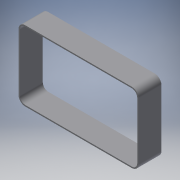
# Autodesk Inventor part: Hub Enclosure Back
Saved by Autodesk Inventor 2018 (Build 220112000, 112)
## iProperties
Created: 2018-03-25
Part Number: Hub Enclosure Back
Material: Generic
Document SubType Name: Modeling
Designer: brutu
Density: 1 g/cm^3
Appearance: Default
Author: brutu
Autodesk Inventor part; units mm, degrees
ref_plane "YZ Plane" through (0, 0, 0) normal (1, 0, 0) x (0, 1, 0)
ref_plane "XZ Plane" through (0, 0, 0) normal (0, 1, 0) x (-1, 0, 0)
ref_plane "XY Plane" through (0, 0, 0) normal (0, 0, 1) x (1, 0, 0)
sketch "Sketch1" plane through (0, 0, 0) normal (0, 0, 1) x (1, 0, 0)
  circle A0 centre (63.1, -31.85) radius 1.905 projected
  circle A1 centre (-63.1, -31.85) radius 1.905 projected
  arc A2 (-66.905, 25.805) -> (-54.205, 38.505) centre (-66.905, 38.505) ccw projected
  line L0 (-54.205, 38.505) -> (-54.205, 51.205) projected
  line L1 (-54.205, 51.205) -> (54.205, 51.205) projected
  line L2 (54.205, 51.205) -> (54.205, 38.505) projected
  arc A3 (54.205, 38.505) -> (66.905, 25.805) centre (66.905, 38.505) ccw projected
  line L3 (66.905, 25.805) -> (92.305, 25.805) projected
  line L4 (92.305, 25.805) -> (92.305, -25.805) projected
  line L5 (92.305, -25.805) -> (66.905, -25.805) projected
  arc A4 (66.905, -25.805) -> (54.205, -38.505) centre (66.905, -38.505) ccw projected
  line L6 (54.205, -38.505) -> (54.205, -51.205) projected
  line L7 (54.205, -51.205) -> (-54.205, -51.205) projected
  line L8 (-54.205, -51.205) -> (-54.205, -38.505) projected
  arc A5 (-54.205, -38.505) -> (-66.905, -25.805) centre (-66.905, -38.505) ccw projected
  line L9 (-66.905, -25.805) -> (-92.305, -25.805) projected
  line L10 (-92.305, -25.805) -> (-92.305, 25.805) projected
  line L11 (-92.305, 25.805) -> (-66.905, 25.805) projected
  circle A6 centre (-63.1, 33.8) radius 1.905 projected
  circle A7 centre (63.1, 33.8) radius 1.905 projected
  line L12 (88.48, 58.38) -> (-88.48, 58.38) projected
  arc A8 (-88.48, 58.38) -> (-99.48, 47.38) centre (-88.48, 47.38) ccw projected
  line L13 (-99.48, 47.38) -> (-99.48, -47.38) projected
  arc A9 (-99.48, -47.38) -> (-88.48, -58.38) centre (-88.48, -47.38) ccw projected
  line L14 (-88.48, -58.38) -> (88.48, -58.38) projected
  arc A10 (88.48, -58.38) -> (99.48, -47.38) centre (88.48, -47.38) ccw projected
  line L15 (99.48, -47.38) -> (99.48, 47.38) projected
  arc A11 (99.48, 47.38) -> (88.48, 58.38) centre (88.48, 47.38) ccw projected
  arc A12 (-88.48, 56.28) -> (-97.38, 47.38) centre (-88.48, 47.38) ccw
  line L16 (-88.48, 56.28) -> (88.48, 56.28)
  arc A13 (97.38, 47.38) -> (88.48, 56.28) centre (88.48, 47.38) ccw
  line L17 (97.38, 47.38) -> (97.38, -47.38)
  arc A14 (88.48, -56.28) -> (97.38, -47.38) centre (88.48, -47.38) ccw
  line L18 (88.48, -56.28) -> (-88.48, -56.28)
  arc A15 (-97.38, -47.38) -> (-88.48, -56.28) centre (-88.48, -47.38) ccw
  line L19 (-97.38, -47.38) -> (-97.38, 47.38)
  point P0 (0, 0)
  dimension "d0" = 2.1
  constraints: 8 end point, 8 point on circle, 4 centre point, 7 other
  measures "d0" distance between parallel lines of L12 L16
extrude "Extrusion1" add sketch "Sketch1" along normal blind 38.1 contours A11 L15 A10 L14 A9 L13 A8 L12
sketch "Sketch2" plane through (-99.48, -47.38, 0) normal (-1, 0, 0) x (0, 0, 1)
  line L0 (0, 79.13) -> (0, 79.13)
  line L1 (12.7, 66.43) -> (12.7, 28.33)
  line L2 (0, 15.63) -> (0, 15.63)
  line L3 (0, 15.63) -> (0, 79.13)
  arc A0 (12.7, 66.43) -> (0, 79.13) centre (0, 66.43) ccw
  arc A1 (0, 15.63) -> (12.7, 28.33) centre (0, 28.33) ccw
  line L4 (0, 94.76) -> (0, 0) projected
  point P0 (0, 47.38)
  point P1 (0, 47.38)
  point P2 (0, 47.38)
  dimension "d3" = 63.5
  dimension "d4" = 12.7
  dimension "d5" = 12.7
  dimension "d6" = 0
  constraints: 8 end point, 4 point on circle, 4 tangent, 2 centre point, 2 midpoint, 2 parallel, 1 coincident, 1 equal radius, 1 horizontal, 1 perpendicular
  measures "d3" distance between parallel lines of L2 L0
  measures "d4" distance between parallel lines of L3 L1
  measures "d5" radius of A0
  measures "d6" distance between parallel lines of L4 L3
extrude "Extrusion2" cut sketch "Sketch2" against normal through all
sketch "Sketch3" plane through (-88.48, 58.38, 0) normal (0, 1, 0) x (1, 0, 0)
  line L0 (37.68, -12.7) -> (139.28, -12.7)
  line L1 (151.98, 0) -> (151.98, 0)
  line L2 (151.98, 0) -> (24.98, 0)
  line L3 (24.98, 0) -> (24.98, 0)
  line L4 (176.96, 0) -> (0, 0) projected
  arc A0 (24.98, 0) -> (37.68, -12.7) centre (37.68, 0) ccw
  arc A1 (139.28, -12.7) -> (151.98, 0) centre (139.28, 0) ccw
  point P0 (88.48, 0)
  point P1 (24.98, -12.7)
  point P2 (151.98, -12.7)
  point P3 (88.48, 0)
  point P4 (88.48, 0)
  point P5 (88.48, 0)
  dimension "d9" = 127
  dimension "d10" = 12.7
  dimension "d11" = 12.7
  constraints: 8 end point, 4 point on circle, 4 point on line, 4 tangent, 3 midpoint, 2 centre point, 2 coincident, 2 parallel, 1 equal radius, 1 horizontal, 1 perpendicular
  measures "d9" distance of point (24.98, -12.7) point (151.98, -12.7)
  measures "d10" distance of L2.end point (24.98, -12.7)
  measures "d11" radius of A0
extrude "Extrusion3" cut sketch "Sketch3" against normal through all
sketch "Sketch4" plane through (0, 0, 38.1) normal (0, 0, 1) x (1, 0, 0)
  line L0 (-88.48, 56.28) -> (88.48, 56.28) projected
  arc A0 (97.38, 47.38) -> (88.48, 56.28) centre (88.48, 47.38) ccw projected
  line L1 (97.38, 47.38) -> (97.38, -47.38) projected
  arc A1 (88.48, -56.28) -> (97.38, -47.38) centre (88.48, -47.38) ccw projected
  line L2 (88.48, -56.28) -> (-88.48, -56.28) projected
  arc A2 (-97.38, -47.38) -> (-88.48, -56.28) centre (-88.48, -47.38) ccw projected
  line L3 (-97.38, -47.38) -> (-97.38, 47.38) projected
  arc A3 (-88.48, 56.28) -> (-97.38, 47.38) centre (-88.48, 47.38) ccw projected
  line L4 (88.48, 58.38) -> (-88.48, 58.38) projected
  arc A4 (-88.48, 58.38) -> (-99.48, 47.38) centre (-88.48, 47.38) ccw projected
  line L5 (-99.48, 47.38) -> (-99.48, -47.38) projected
  arc A5 (-99.48, -47.38) -> (-88.48, -58.38) centre (-88.48, -47.38) ccw projected
  line L6 (-88.48, -58.38) -> (88.48, -58.38) projected
  arc A6 (88.48, -58.38) -> (99.48, -47.38) centre (88.48, -47.38) ccw projected
  line L7 (99.48, -47.38) -> (99.48, 47.38) projected
  arc A7 (99.48, 47.38) -> (88.48, 58.38) centre (88.48, 47.38) ccw projected
  point P0 (0, 0)
body "Solid1"
